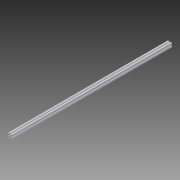
# Autodesk Inventor part: 8020_40
Saved by Autodesk Inventor 2011 SP1 (Build 150282100, 282)
## iProperties
Created: 2013-01-16
Part Number: 8020_40
Document SubType Name: Modeling
Designer: 917788
Density: 1 g/cm^3
Author: 917788
Autodesk Inventor part; units mm, degrees
ref_plane "YZ Plane" through (0, 0, 0) normal (1, 0, 0) x (0, 1, 0)
ref_plane "XZ Plane" through (0, 0, 0) normal (0, 1, 0) x (-1, 0, 0)
ref_plane "XY Plane" through (0, 0, 0) normal (0, 0, 1) x (1, 0, 0)
sketch "Sketch1" plane through (0, 0, 0) normal (0, 0, 1) x (1, 0, 0)
  line L0 (0, 9.525) -> (3.175, 9.525)
  line L1 (3.175, 9.525) -> (3.175, 4.7625)
  line L2 (3.175, 20.6375) -> (3.175, 15.875)
  line L3 (3.175, 15.875) -> (0, 15.875)
  line L4 (7.9375, 15.875) -> (7.9375, 9.525)
  line L5 (25.4, 15.875) -> (22.225, 15.875)
  line L6 (22.225, 15.875) -> (22.225, 20.6375)
  line L7 (22.225, 20.6375) -> (17.4625, 15.875)
  line L8 (17.4625, 15.875) -> (17.4625, 9.525)
  line L9 (17.4625, 9.525) -> (22.225, 4.7625)
  line L10 (22.225, 4.7625) -> (22.225, 9.525)
  line L11 (22.225, 9.525) -> (25.4, 9.525)
  line L12 (25.4, 15.875) -> (25.4, 25.4)
  line L13 (25.4, 9.525) -> (25.4, 0)
  line L14 (12.7, 12.7) -> (25.4, 25.4)
  line L15 (12.7, 12.7) -> (0, 25.4)
  line L16 (12.7, 12.7) -> (0, 0)
  line L17 (12.7, 12.7) -> (25.4, 0)
  line L18 (0, 25.4) -> (9.525, 25.4)
  line L19 (9.525, 25.4) -> (9.525, 22.225)
  line L20 (9.525, 22.225) -> (4.7625, 22.225)
  line L21 (4.7625, 22.225) -> (9.525, 17.4625)
  line L22 (9.525, 17.4625) -> (15.875, 17.4625)
  line L23 (15.875, 17.4625) -> (20.6375, 22.225)
  line L24 (20.6375, 22.225) -> (15.875, 22.225)
  line L25 (15.875, 22.225) -> (15.875, 25.4)
  line L26 (15.875, 25.4) -> (25.4, 25.4)
  line L27 (0, 0) -> (9.525, 0)
  line L28 (9.525, 0) -> (9.525, 3.175)
  line L29 (9.525, 3.175) -> (4.7625, 3.175)
  line L30 (4.7625, 3.175) -> (9.525, 7.9375)
  line L31 (9.525, 7.9375) -> (15.875, 7.9375)
  line L32 (15.875, 7.9375) -> (20.6375, 3.175)
  line L33 (20.6375, 3.175) -> (15.875, 3.175)
  line L34 (15.875, 3.175) -> (15.875, 0)
  line L35 (15.875, 0) -> (25.4, 0)
  line L36 (0, 25.4) -> (0, 15.875)
  line L37 (0, 9.525) -> (0, 0)
  line L38 (7.9375, 9.525) -> (3.175, 4.7625)
  line L39 (7.9375, 15.875) -> (3.175, 20.6375)
  dimension "d1" = 25.4
  dimension "d5" = 3.175
  dimension "d6" = 4.7625
  dimension "d7" = 4.7625
  dimension "d9" = 6.35
  dimension "d10" = 3.175
  dimension "d11" = 4.7625
  dimension "d12" = 4.7625
  dimension "d13" = 3.175
  dimension "d15" = 9.525
  dimension "d16" = 3.175
  dimension "d17" = 4.7625
  dimension "d18" = 6.35
  dimension "d19" = 4.7625
  dimension "d20" = 9.525
  dimension "d21" = 3.175
  dimension "d22" = 4.7625
  dimension "d23" = 6.35
  dimension "d24" = 4.7625
  constraints: 80 end point, 16 perpendicular, 6 parallel, 5 collinear, 2 point on line
  measures "d1" distance of L12.end L13.end
  measures "d5" distance of L2.end L3.end
  measures "d6" distance of L2.start L2.end
  measures "d7" distance of L0.end L1.end
  measures "d9" distance of L4.start L4.end
  measures "d10" distance of L5.start L5.end
  measures "d11" distance of L5.end L6.end
  measures "d12" distance of L9.end L10.end
  measures "d13" distance of L10.end L11.end
  measures "d15" distance of L15.end L18.end
  measures "d16" distance of L18.end L19.end
  measures "d17" distance of L19.end L20.end
  measures "d18" distance of L21.end L22.end
  measures "d19" distance of L23.end L24.end
  measures "d20" distance of L16.end L27.end
  measures "d21" distance of L27.end L28.end
  measures "d22" distance of L28.end L29.end
  measures "d23" distance of L30.end L31.end
  measures "d24" distance of L32.end L33.end
extrude "Extrusion1" add sketch "Sketch1" against normal blind 1016
body "Solid1"
